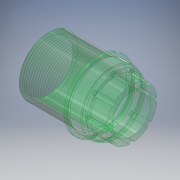
# Autodesk Inventor part: entraineur
Saved by Autodesk Inventor 2018.1 (Build 221171000, 171)
## iProperties
Created: 2022-05-13
Part Number: entraineur
Material: Generic
Document SubType Name: Modeling
Designer: Bureau
Density: 1 g/cm^3
Appearance: Default
Author: Bureau
Autodesk Inventor part; units mm, degrees
ref_plane "YZ Plane" through (0, 0, 0) normal (1, 0, 0) x (0, 1, 0)
ref_plane "XZ Plane" through (0, 0, 0) normal (0, 1, 0) x (-1, 0, 0)
ref_plane "XY Plane" through (0, 0, 0) normal (0, 0, 1) x (1, 0, 0)
sketch "Sketch1" plane through (0, 0, 0) normal (0, 0, 1) x (1, 0, 0)
  line L0 (0, 0) -> (30, 0)
  line L1 (32, 20) -> (25, 20)
  line L2 (25, 20) -> (25, 22)
  line L3 (0, 16) -> (31, 16)
  line L4 (31, 16) -> (31, 12.6)
  line L5 (31, 12.6) -> (31, 12.6)
  line L6 (0, 19) -> (23, 19)
  line L7 (23, 19) -> (23, 22)
  line L8 (23, 22) -> (25, 22)
  line L9 (0, 19) -> (-9, 19)
  line L10 (-9, 19) -> (-9, 16)
  line L11 (-9, 16) -> (0, 16)
  line L12 (31, 12.6) -> (45, 12.6)
  line L13 (45, 12.6) -> (45, 16.5)
  line L14 (32, 20) -> (32, 19)
  line L15 (32, 19) -> (35, 19)
  line L16 (35, 19) -> (35, 16.5)
  line L17 (35, 16.5) -> (45, 16.5)
  dimension "d5" = 2
  dimension "d8" = 16
  dimension "d13" = 3
  dimension "d14" = 23
  dimension "d32" = 9
  dimension "d33" = 14
  dimension "d34" = 40
  dimension "d36" = 16.5
  dimension "d60" = 54
  dimension "d61" = 2
  dimension "d62" = 7
  dimension "d63" = 3
  dimension "d64" = 10
  constraints: 36 end point, 8 perpendicular, 4 horizontal, 2 vertical
  measures "d5" distance of L1.end L2.end
  measures "d8" distance of L0.start L3.start
  measures "d13" distance of L3.start L6.start
  measures "d14" distance of L6.start L6.end
  measures "d32" distance of L6.start L9.end
  measures "d33" distance of L4.end L12.end
  measures "d34" distance of L3.end L10.end
  measures "d36" distance from line of L0 L13.end
  measures "d60" horizontal distance of L13.end L9.end
  measures "d61" distance of L7.end L2.end
  measures "d62" distance of L1.start L1.end
  measures "d63" distance of L14.end L15.end
  measures "d64" distance of L16.end L13.end
revolve "Revolution1" add sketch "Sketch1" angle 360 about axis through (0, 0, 0) along (1, 0, 0)
thread "Thread2" size "M38x1.5" class "6g" standard "ANSI Metric M Profile" full length
thread "Thread3" size "M33x1" class "6g" standard "ANSI Metric M Profile" length 6
sketch "Sketch4" plane through (45, 0, 0) normal (1, 0, 0) x (0, 0, -1)
  circle A0 centre (0, 0) radius 16.5 projected
  circle A1 centre (0, 16.5) radius 1.5
  circle A2 centre (-11.6673, 11.6673) radius 1.5
  circle A3 centre (-16.5, 0) radius 1.5
  circle A4 centre (-11.6673, -11.6673) radius 1.5
  circle A5 centre (0, -16.5) radius 1.5
  circle A6 centre (11.6673, -11.6673) radius 1.5
  circle A7 centre (16.5, 0) radius 1.5
  circle A8 centre (11.6673, 11.6673) radius 1.5
  dimension "d51" = 3
  dimension "d54" = 360
  constraints: 8 centre point, 1 vertical alignment, 18 other
  measures "d51" diameter of A1
extrude "Extrusion3" cut sketch "Sketch4" against normal blind 12 contours A0 A7 | A0 A7 | A8 A0 | A0 A8 | A6 A0 | A0 A6 | A1 A0 | A0 A1 | A5 A0 | A0 A5 | A2 A0 | A0 A2 | A4 A0 | A0 A4 | A3 A0 | A0 A3
body "Solid1"
